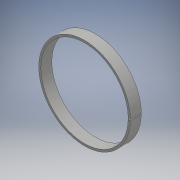
# Autodesk Inventor part: valset ring
Saved by Autodesk Inventor 2018 (Build 220112000, 112)
## iProperties
Created: 2019-10-04
Part Number: valset ring
Material: S235JR
Document SubType Name: Sheet Metal
Designer: gust3763
Density: 7.85 g/cm^3
Appearance: Light Gray
Flat Pattern Width: 2.5 cm
Flat Pattern Length: 64.0358 cm
Flat Pattern Area: 160.089 cm^2
Sheet Metal Rule: Default_mm
Sheet Metal Width: 25,000 mm
Sheet Metal Length: 640,358 mm
Sheet Metal Area: 16008,945 mm^2
Author: gust3763
Autodesk Inventor part; units mm, degrees
ref_plane "YZ Plane" through (0, 0, 0) normal (1, 0, 0) x (0, 1, 0)
ref_plane "XZ Plane" through (0, 0, 0) normal (0, 1, 0) x (-1, 0, 0)
ref_plane "XY Plane" through (0, 0, 0) normal (0, 0, 1) x (1, 0, 0)
sketch "Sketch1" plane through (0, 0, 0) normal (0, 0, 1) x (1, 0, 0)
  line L0 (0, 0) -> (0, 18.9343)
  line L1 (100, 0) -> (105, 0)
  line L2 (105, 0) -> (105, 25)
  line L3 (105, 25) -> (100, 25)
  line L4 (100, 25) -> (100, 0)
  dimension "d0" = 5
  dimension "d1" = 200
  dimension "d2" = 25
  constraints: 10 end point, 2 horizontal, 2 parallel, 1 perpendicular, 1 vertical
  measures "d0" distance of L1.start L1.end
  measures "d1" diameter of L4 L0
  measures "d2" distance between parallel lines of L3 L1
revolve "Revolution1" add sketch "Sketch1" angle 359 about axis through (0, 0, 0) along (0, -1, 0)
sketch "Sketch2" plane through (0, 0, 0) normal (1, 0, 0) x (0, 1, 0)
  line L0 (25, 105) -> (25, -105) projected
  line L1 (0, 105) -> (0, -105) projected
  circle A0 centre (12.5, 0) radius 5
  point P0 (0, 0)
  point P1 (25, 0)
  point P2 (25, -1.8325)
  point P3 (0, -1.8325)
  dimension "d4" = 10
  dimension "d5" = 210
  dimension "d6" = 25
  dimension "d7" = 12.5
  dimension "d8" = 105
  constraints: 1 centre point
  measures "d4" diameter of A0
  measures "d5" distance of L0.start L0.end
  measures "d6" distance between parallel lines of L1 L0
  measures "d7" distance from line of A0.centre L1
  measures "d8" vertical distance of A0.centre L0.end
extrude "Extrusion1" [suppressed]
equation "\"d7\" = 0.5 * d6"
equation "\"d8\" = 0.5 * d5"
equation "\"BendRadius\" = Thickness"
equation "\"BendReliefWidth\" = Thickness"
equation "\"BendReliefDepth\" = 0.5 * Thickness"
equation "\"TransitionRadius\" = BendRadius"
equation "\"JacobiRadiusSize\" = BendRadius"
equation "\"GapSize\" = Thickness"
equation "\"Thickness\" = 5"
body "Solid1"
